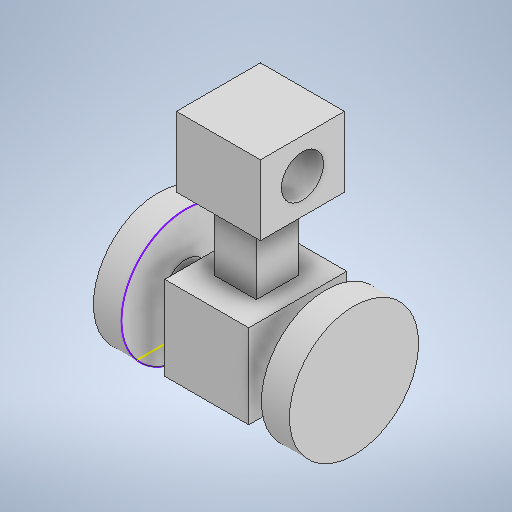
# Autodesk Inventor part: Part4_remodified
Saved by Autodesk Inventor 2025.2 (Build 292293000, 293)
## iProperties
Created: 2025-01-27
Part Number: Part4_remodified
Material: Generic
Document SubType Name: Modeling
Designer: ckond
Density: 1 g/cm^3
Appearance: Default
Author: ckond
Autodesk Inventor part; units mm, degrees
ref_plane "YZ Plane" through (0, 0, 0) normal (1, 0, 0) x (0, 1, 0)
ref_plane "XZ Plane" through (0, 0, 0) normal (0, 1, 0) x (-1, 0, 0)
ref_plane "XY Plane" through (0, 0, 0) normal (0, 0, 1) x (1, 0, 0)
sketch "Sketch1" plane through (0, 0, 0) normal (0, 0, 1) x (1, 0, 0)
  line L0 (-15, 12.5) -> (15, 12.5)
  line L1 (15, 12.5) -> (15, -12.5)
  line L2 (15, -12.5) -> (-15, -12.5)
  line L3 (-15, -12.5) -> (-15, 12.5)
  line L4 (-15, 12.5) -> (15, -12.5) construction
  line L5 (15, 12.5) -> (-15, -12.5) construction
  point P0 (0, 0)
  dimension "d0" = 30
  dimension "d1" = 25
  constraints: 12 end point, 2 midpoint, 2 parallel, 1 horizontal, 1 perpendicular
  measures "d0" distance of L1.end L2.end
  measures "d1" distance of L0.end L1.end
extrude "Extrusion1" add sketch "Sketch1" along normal blind 30
sketch "Sketch2" plane through (15, -12.5, 0) normal (1, 0, 0) x (0, 0, -1)
  circle A0 centre (-15.0077, 12.5) radius 7.5
  point P0 (0, 12.5)
  dimension "d4" = 15
  constraints: 1 centre point
  measures "d4" diameter of A0
extrude "Extrusion2" cut sketch "Sketch2" against normal through all
sketch "Sketch3" plane through (-15, -12.5, 0) normal (0, -1, 0) x (1, 0, 0)
  line L0 (7.5, 23.9638) -> (22.5, 23.9638)
  line L1 (22.5, 23.9638) -> (22.5, 8.9638)
  line L2 (22.5, 8.9638) -> (7.5, 8.9638)
  line L3 (7.5, 8.9638) -> (7.5, 23.9638)
  line L4 (7.5, 23.9638) -> (22.5, 8.9638) construction
  line L5 (22.5, 23.9638) -> (7.5, 8.9638) construction
  point P0 (15, 0)
  point P1 (15, 16.4638)
  dimension "d7" = 15
  dimension "d8" = 15
  constraints: 12 end point, 2 midpoint, 2 parallel, 1 horizontal, 1 perpendicular
  measures "d7" distance of L1.end L2.end
  measures "d8" distance of L0.end L1.end
extrude "Extrusion3" add sketch "Sketch3" along normal blind 25
sketch "Sketch4" plane through (-15, -37.5, 0) normal (0, -1, 0) x (1, 0, 0)
  line L0 (-0.1247, 34.0483) -> (29.8753, 34.0483)
  line L1 (29.8753, 34.0483) -> (29.8753, -0.9517)
  line L2 (29.8753, -0.9517) -> (-0.1247, -0.9517)
  line L3 (-0.1247, -0.9517) -> (-0.1247, 34.0483)
  line L4 (-0.1247, 34.0483) -> (29.8753, -0.9517) construction
  line L5 (29.8753, 34.0483) -> (-0.1247, -0.9517) construction
  point P0 (15, 0)
  point P1 (14.8753, 16.5483)
  dimension "d11" = 30
  dimension "d12" = 35
  constraints: 12 end point, 2 midpoint, 2 parallel, 1 horizontal, 1 perpendicular
  measures "d11" distance of L1.end L2.end
  measures "d12" distance of L2.end L0.start
extrude "Extrusion4" add sketch "Sketch4" along normal blind 30
sketch "Sketch5" plane through (-15.1247, -37.5, -0.9517) normal (-1, 0, 0) x (0, 0, 1)
  circle A0 centre (17.4156, -15.0883) radius 7.5
  point P0 (0.9517, 37.5)
  dimension "d15" = 15
  constraints: 1 centre point
  measures "d15" diameter of A0
extrude "Extrusion5" add sketch "Sketch5" along normal blind 10
sketch "Sketch6" plane through (14.8753, -37.5, 34.0483) normal (1, 0, 0) x (0, 0, -1)
  circle A0 centre (17.5844, -15.0883) radius 7.5 projected
  circle A1 centre (17.5844, -15.0883) radius 7.5
  point P0 (34.0483, 37.5)
  constraints: 1 centre point, 1 coincident
extrude "Extrusion6" add sketch "Sketch6" along normal blind 10
sketch "Sketch7" plane through (-25.1247, -52.5883, 16.4638) normal (-1, 0, 0) x (0, 0, 1)
  line L0 (-17.4156, -14.9117) -> (17.5844, -14.9117) projected
  circle A0 centre (0, 0) radius 23.0558
  point P0 (-16.4638, 52.5883)
  constraints: 3 other
extrude "Extrusion7" add sketch "Sketch7" along normal blind 10
sketch "Sketch8" plane through (24.8753, -52.5883, 16.4638) normal (1, 0, 0) x (0, 0, -1)
  circle A0 centre (0, 0) radius 7.5 projected
  circle A1 centre (0, 0) radius 23.0558 projected
  circle A2 centre (0, 0) radius 23.056
  point P0 (16.4638, 52.5883)
  dimension "d22" = 46.112
  constraints: 1 centre point, 1 coincident
  measures "d22" diameter of A2
extrude "Extrusion8" add sketch "Sketch8" along normal blind 10 contours A0 | A1
body "Solid1"
